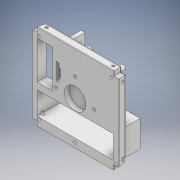
# Autodesk Inventor part: boxbase_solar_esp8285
Saved by Autodesk Inventor 2017 (Build 210142000, 142)
## iProperties
Created: 2018-12-11
Part Number: boxbase_solar_esp8285
Material: ABS Plastic
Document SubType Name: Modeling
Designer: simulator
Density: 1.06 g/cm^3
Appearance: Smooth - White
Mass: 72.9733 g
Surface Area: 351.505 cm^2
Volume: 68.8428 cm^3
Author: simulator
## iProperties of the stored document boxbase_solar_esp8285_3DPrint.ipt
Created: 2019-04-02
Part Number: boxbase_solar_esp8285_3DPrint
Material: Generic
Document SubType Name: Modeling
Designer: simulator
Density: 1 g/cm^3
Appearance: Default
Author: simulator
Autodesk Inventor part; units mm, degrees
ref_plane "YZ Plane" through (0, 0, 0) normal (1, 0, 0) x (0, 1, 0)
sketch "Sketch1" plane through (0, 0, 0) normal (0, 1, 0) x (-1, 0, 0)
  circle A0 centre (45, -45) radius 1.5
  circle A1 centre (-45, 45) radius 1.5
  circle A2 centre (-45, -45) radius 1.5
  circle A3 centre (45, 45) radius 1.5
  line L0 (-50, -50) -> (50, -50)
  line L1 (50, 50) -> (50, -50)
  line L2 (-50, 50) -> (50, 50)
  line L3 (-50, -50) -> (-50, 50)
  line L4 (40, -45) -> (-40, -45)
  line L5 (-40, -40) -> (-40, -45)
  line L6 (-45, -40) -> (-40, -40)
  line L7 (-45, -40) -> (-45, 40)
  line L8 (-40, 40) -> (-45, 40)
  line L9 (-40, 45) -> (-40, 40)
  line L10 (-40, 45) -> (40, 45)
  line L11 (40, 40) -> (40, 45)
  line L12 (45, 40) -> (40, 40)
  line L13 (45, 40) -> (45, -40)
  line L14 (40, -40) -> (45, -40)
  line L15 (40, -45) -> (40, -40)
  point P0 (0, 0)
  point P1 (0, 0)
  constraints: 32 end point, 4 centre point
extrude "Extrusion1" add sketch "Sketch1" along normal blind 10 contours L4 L5 L6 L7 L8 L9 L10 L11 L12 L13 L14 L15
sketch "Sketch2" plane through (45, 0, 40) normal (1, 0, 0) x (0, 0, -1)
  line L0 (0, 10) -> (80, 10)
  line L1 (0, 0) -> (0, 10)
  line L2 (0, 0) -> (80, 0)
  line L3 (80, 10) -> (80, 0)
  circle A0 centre (5, 5) radius 1.5
  circle A1 centre (75, 5) radius 1.5
  point P0 (40, 0)
  point P1 (40, 0)
  constraints: 8 end point, 2 centre point, 2 coincident
hole "Hole1" at (45, 5, 35) at (45, 5, -35) direction (-1, 0, 0) diameter 3 depth 8 tip angle 118
sketch "Sketch3" plane through (-40, 0, 45) normal (0, 0, 1) x (1, 0, 0)
  line L0 (0, 10) -> (80, 10)
  line L1 (0, 0) -> (0, 10)
  line L2 (0, 0) -> (80, 0)
  line L3 (80, 10) -> (80, 0)
  circle A0 centre (5, 5) radius 1.5
  circle A1 centre (75, 5) radius 1.5
  point P0 (40, 0)
  point P1 (40, 0)
  constraints: 8 end point, 2 centre point, 2 coincident
hole "Hole2" at (-35, 5, 45) at (35, 5, 45) direction (0, 0, -1) diameter 3 depth 8 tip angle 118
sketch "Sketch4" plane through (0, 10, 0) normal (0, 1, 0) x (1, 0, 0)
  point P0 (0, 0)
sketch "Sketch5" plane through (40, 0, -45) normal (0, 0, -1) x (-1, 0, 0)
  line L0 (0, 10) -> (80, 10)
  line L1 (0, 0) -> (0, 10)
  line L2 (0, 0) -> (80, 0)
  line L3 (80, 10) -> (80, 0)
  circle A0 centre (5, 5) radius 1.5
  circle A1 centre (75, 5) radius 1.5
  circle A2 centre (75, 5) radius 1.5 projected
  point P0 (40, 0)
  point P1 (40, 0)
  constraints: 8 end point, 2 centre point, 2 coincident
hole "Hole3" at (-35, 5, -45) at (35, 5, -45) direction (0, 0, 1) diameter 3 depth 8 tip angle 118
sketch "Sketch6" plane through (-45, 0, -40) normal (-1, 0, 0) x (0, 0, 1)
  line L0 (0, 10) -> (80, 10)
  line L1 (0, 0) -> (0, 10)
  line L2 (0, 0) -> (80, 0)
  line L3 (80, 10) -> (80, 0)
  circle A0 centre (5, 5) radius 1.5
  circle A1 centre (75, 5) radius 1.5
  circle A2 centre (5, 5) radius 1.5 projected
  circle A3 centre (75, 5) radius 1.5 projected
  point P0 (40, 0)
  point P1 (40, 0)
  constraints: 8 end point, 2 centre point, 2 coincident
hole "Hole4" at (-45, 5, -35) at (-45, 5, 35) direction (1, 0, 0) diameter 3 depth 8 tip angle 118
chamfer "Chamfer1" distance 1 distance2 9 1 edges at (45, 10, 0)
chamfer "Chamfer2" distance 1 distance2 9 1 edges at (42, 10, 40) measured on face at (42, 10, 39.5)
chamfer "Chamfer3" distance 1 distance2 9 2 edges at (40, 10, 39.5) (40, 10, 42.5) measured on face at (39.5, 10, 42.5) measured on face at (39.5, 10, 39.5)
chamfer "Chamfer4" distance 1 distance2 9 1 edges at (-0.5, 10, 45)
chamfer "Chamfer5" distance 1 distance2 9 1 edges at (-40, 10, 42) measured on face at (-39.5, 10, 42)
chamfer "Chamfer6" distance 1 distance2 9 2 edges at (-39.5, 10, 40) (-42.5, 10, 40) measured on face at (-39.5, 10, 39.5) measured on face at (-42.5, 10, 39.5)
chamfer "Chamfer7" distance 1 distance2 9 1 edges at (-45, 10, -0.5)
chamfer "Chamfer8" distance 1 distance2 9 1 edges at (-42, 10, -40) measured on face at (-42, 10, -39.5)
chamfer "Chamfer9" distance 1 distance2 9 2 edges at (-40, 10, -39.5) (-40, 10, -42.5) measured on face at (-39.5, 10, -39.5) measured on face at (-39.5, 10, -42.5)
chamfer "Chamfer10" distance 1 distance2 9 1 edges at (0.5, 10, -45)
chamfer "Chamfer11" distance 1 distance2 9 1 edges at (40, 10, -42) measured on face at (39.5, 10, -42)
chamfer "Chamfer12" distance 1 distance2 9 2 edges at (39.5, 10, -40) (42, 10, -40) measured on face at (42, 10, -39.5) measured on face at (39.5, 10, -39.5)
sketch "Sketch21" plane through (0, 0, 0) normal (0, -1, 0) x (1, 0, 0)
  line L0 (-40, 36) -> (40, 36)
  line L1 (40, 36) -> (40, 12)
  line L2 (40, 12) -> (-40, 12)
  line L3 (-40, 12) -> (-40, 36)
  point P0 (0, 0)
  dimension "d153" = 80
  dimension "d154" = 24
  dimension "d155" = 40
  dimension "d156" = 12
  constraints: 8 end point, 2 parallel, 1 horizontal
  measures "d153" distance of L1.end L2.end
  measures "d154" distance of L0.end L1.end
  measures "d155" distance from line of L1 point (0, 0)
  measures "d156" distance from line of L2 point (0, 0)
sketch "Sketch24" plane through (0, 10, 0) normal (0, 1, 0) x (1, 0, 0)
  line L0 (28.9892, 33.853) -> (-5.0108, 33.853)
  line L1 (-5.0108, 33.853) -> (-5.0108, -0.147)
  line L2 (-5.0108, -0.147) -> (28.9892, -0.147)
  line L3 (28.9892, -0.147) -> (28.9892, 33.853)
  line L4 (32.9892, 37.853) -> (-9.0108, 37.853)
  line L5 (-9.0108, 37.853) -> (-9.0108, -4.147)
  line L6 (-9.0108, -4.147) -> (32.9892, -4.147)
  line L7 (32.9892, -4.147) -> (32.9892, 37.853)
  line L8 (35, -4) -> (1, -4)
  line L9 (1, -4) -> (1, -38)
  line L10 (1, -38) -> (35, -38)
  line L11 (35, -38) -> (35, -4)
  line L12 (-19.3264, -7.8069) -> (-37.3264, -7.8069)
  line L13 (-37.3264, -7.8069) -> (-37.3264, -32.8069)
  line L14 (-37.3264, -32.8069) -> (-19.3264, -32.8069)
  line L15 (-19.3264, -32.8069) -> (-19.3264, -7.8069)
  line L16 (-34.8264, -7.8069) -> (-21.8264, -7.8069)
  line L17 (44, 39) -> (44, -39) projected
  line L18 (39, -44) -> (-39, -44) projected
  line L19 (45, -40) -> (45, 40) projected
  line L20 (-40, -45) -> (40, -45) projected
  circle A0 centre (1, -4) radius 3
  circle A1 centre (35, -4) radius 3
  circle A2 centre (1, -38) radius 3
  circle A3 centre (35, -38) radius 3
  point P0 (0, 0)
  dimension "d169" = 34
  dimension "d170" = 34
  dimension "d171" = 42
  dimension "d172" = 34
  dimension "d173" = 34
  dimension "d174" = 18
  dimension "d175" = 25
  dimension "d176" = 13
  dimension "d177" = 2.5
  dimension "d215" = 10
  dimension "d216" = 7
  dimension "d217" = 6
  dimension "d218" = 6
  dimension "d219" = 6
  dimension "d220" = 6
  constraints: 34 end point, 10 coincident, 8 parallel, 4 centre point, 4 perpendicular, 3 horizontal, 2 point on line, 3 other
  measures "d169" distance of L2.end L1.end
  measures "d170" distance of L1.end L0.end
  measures "d171" distance of L6.end L4.start
  measures "d172" distance of L10.end L9.end
  measures "d173" distance of L9.end L8.end
  measures "d174" distance of L14.end L13.end
  measures "d175" distance of L13.end L12.end
  measures "d176" distance of L16.start L16.end
  measures "d177" distance from line of L15 L16.end
  measures "d215" distance between parallel lines of L11 L19
  measures "d216" distance between parallel lines of L10 L20
  measures "d217" diameter of A0
  measures "d218" diameter of A1
  measures "d219" diameter of A2
  measures "d220" diameter of A3
sketch "Sketch25" plane through (0, 10, 0) normal (0, 1, 0) x (1, 0, 0)
  line L0 (-40, 36) -> (40, 36)
  line L1 (40, 36) -> (40, 12)
  line L2 (40, 12) -> (-40, 12)
  line L3 (-40, 12) -> (-40, 36)
  line L4 (42, 10) -> (42, 38)
  line L5 (42, 38) -> (-42, 38)
  line L6 (-42, 38) -> (-42, 10)
  line L7 (-42, 10) -> (42, 10)
  point P0 (0, 0)
  point P1 (0, 0)
  dimension "d178" = 80
  dimension "d179" = 24
  dimension "d180" = 40
  dimension "d181" = 12
  dimension "d182" = 2
  constraints: 16 end point, 4 parallel, 1 horizontal, 3 other
  measures "d178" distance of L1.end L2.end
  measures "d179" distance of L0.end L1.end
  measures "d180" distance from line of L1 point (0, 0)
  measures "d181" distance from line of L2 point (0, 0)
  measures "d182" distance between parallel lines of L1 L4
extrude "Extrusion19" add sketch "Sketch25" along normal blind 14
sketch "Sketch26" plane through (0, 24, 0) normal (0, 1, 0) x (1, 0, 0)
  line L0 (40, 36) -> (40, 12) projected
  line L1 (42, 10) -> (42, 38) projected
  line L2 (40, 36) -> (40, 12) projected
  line L3 (40, 12) -> (-40, 12) projected
  line L4 (-40, 12) -> (-40, 36) projected
  line L5 (-40, 36) -> (40, 36) projected
  line L6 (42, 10) -> (42, 38) projected
  line L7 (42, 38) -> (-42, 38) projected
  line L8 (-42, 38) -> (-42, 10) projected
  line L9 (-42, 10) -> (42, 10) projected
  point P0 (0, 0)
extrude "Extrusion20" add sketch "Sketch26" along normal blind 2 contours L0 L3 L4 L5 | L9 L8 L7 L1
sketch "Sketch27" plane through (0, 0, 0) normal (0, -1, 0) x (1, 0, 0)
  line L0 (40, -36) -> (40, -12) projected
  line L1 (40, -12) -> (-40, -12) projected
  line L2 (-40, -36) -> (40, -36) projected
  line L3 (-40, -12) -> (-40, -36) projected
  point P0 (0, 0)
extrude "Extrusion21" cut sketch "Sketch27" against normal blind 24
sketch "Sketch28" plane through (0, 26, 0) normal (0, 1, 0) x (1, 0, 0)
  line L0 (-37, 33) -> (-12, 33)
  line L1 (-12, 33) -> (-12, 15)
  line L2 (-12, 15) -> (-37, 15)
  line L3 (-37, 15) -> (-37, 33)
  line L4 (-12, 17.5) -> (-12, 30.5)
  line L5 (-42, 38) -> (-42, 10) projected
  line L6 (42, 38) -> (-42, 38) projected
  circle A0 centre (-12, 30.5) radius 3
  circle A1 centre (-12, 17.5) radius 3
  line L7 (0, 36.4802) -> (32, 36.4802)
  line L8 (32, 36.4802) -> (32, 4.4802)
  line L9 (32, 4.4802) -> (0, 4.4802)
  line L10 (0, 4.4802) -> (0, 36.4802)
  point P0 (0, 0)
  dimension "d189" = 25
  dimension "d190" = 18
  dimension "d191" = 13
  dimension "d192" = 2.5
  dimension "d193" = 5
  dimension "d194" = 5
  dimension "d195" = 6
  dimension "d196" = 6
  dimension "d213" = 32
  dimension "d214" = 32
  constraints: 18 end point, 4 coincident, 4 parallel, 2 centre point, 2 horizontal, 2 perpendicular, 2 point on line
  measures "d189" distance of L1.end L2.end
  measures "d190" distance of L0.end L1.end
  measures "d191" distance of L4.start L4.end
  measures "d192" distance of L4.start L1.end
  measures "d193" distance between parallel lines of L5 L3
  measures "d194" distance between parallel lines of L6 L0
  measures "d195" diameter of A0
  measures "d196" diameter of A1
  measures "d213" distance of L8.end L9.end
  measures "d214" distance of L7.end L8.end
extrude "Extrusion22" add sketch "Sketch28" along normal blind 5 contours A0 L1 L0 | L0 L1 A0 | A1 L1 L2 | L2 L1 A1
sketch "Sketch29" plane through (-12, 31, -17.5) normal (0, 1, 0) x (1, 0, 0)
  circle A0 centre (0, 13) radius 3 projected
  circle A1 centre (0, 0) radius 3 projected
  point P0 (12, -17.5)
  constraints: 2 coincident
hole "Hole6" at (-12, 31, -17.5) at (-12, 31, -30.5) direction (0, -1, 0) diameter 3 depth 8 tip angle 118
sketch "Sketch30" plane through (0, 26, 0) normal (0, 1, 0) x (1, 0, 0)
  circle A0 centre (-12, 17.5) radius 3 projected
  circle A1 centre (-12, 30.5) radius 3 projected
  line L0 (42, 10) -> (42, 38) projected
  line L1 (42, 38) -> (-42, 38) projected
  line L2 (-42, 38) -> (-42, 10) projected
  line L3 (-42, 10) -> (42, 10) projected
  line L4 (42, 10) -> (42, 38) projected
  line L5 (-42, 10) -> (42, 38)
  point P0 (0, 0)
  point P1 (0, 24)
  constraints: 2 end point, 1 midpoint
hole "Hole7" at (0, 26, -24) direction (0, -1, 0) diameter 3 depth 8 tip angle 118
extrude "Extrusion23" add sketch "Sketch24" along normal blind 5 contours A1 L11 L8 L7 | L7 L8 A1 | L8 L11 A1 L6 L7 | L7 L6 A1 L8 | A0 L8 L9 L6 | L6 L9 A0 | A0 L6 L9 L8 | L6 A0 L9 | A3 L10 L11 | L11 L10 A3 | A2 L10 L9 | L9 L10 A2
sketch "Sketch31" plane through (1, 15, 4) normal (0, 1, 0) x (1, 0, 0)
  circle A0 centre (0, 0) radius 3 projected
  circle A1 centre (34, 0) radius 3 projected
  circle A2 centre (0, -34) radius 3 projected
  circle A3 centre (34, -34) radius 3 projected
  circle A4 centre (0, 0) radius 3 projected
  circle A5 centre (34, 0) radius 3 projected
  point P0 (-1, 4)
  constraints: 4 coincident
hole "Hole8" at (1, 15, 4) at (1, 15, 38) at (35, 15, 38) at (35, 15, 4) direction (0, -1, 0) diameter 3 depth 8 tip angle 118
sketch "Sketch32" plane through (0, 10, 0) normal (0, 1, 0) x (1, 0, 0)
  line L0 (-30, 2) -> (-25, 2)
  line L1 (-25, 2) -> (-25, -30)
  line L2 (-25, -30) -> (-30, -30)
  line L3 (-30, -30) -> (-30, 2)
  line L4 (-45, 40) -> (-45, -40) projected
  line L5 (-40, -45) -> (40, -45) projected
  point P0 (0, 0)
  dimension "d230" = 5
  dimension "d231" = 32
  dimension "d232" = 15
  dimension "d233" = 15
  constraints: 8 end point, 2 parallel, 1 horizontal, 1 perpendicular
  measures "d230" distance of L1.end L2.end
  measures "d231" distance of L0.end L1.end
  measures "d232" distance between parallel lines of L3 L4
  measures "d233" distance between parallel lines of L2 L5
ref_plane "Work Plane1" through (-25, 10, 30) normal (1, 0, 0) x (0, 0, -1)
sketch "Sketch35" plane through (0, 10, 0) normal (0, 1, 0) x (1, 0, 0)
  line L0 (42, 10) -> (-42, 10) projected
  line L1 (-42, 10) -> (-42, 38) projected
  line L2 (-42, 38) -> (42, 38) projected
  line L3 (42, 38) -> (42, 10) projected
  line L4 (39, 39) -> (44, 39) projected
  line L5 (39, 44) -> (39, 39) projected
  line L6 (-39, 44) -> (39, 44) projected
  line L7 (-39, 39) -> (-39, 44) projected
  line L8 (-44, 39) -> (-39, 39) projected
  line L9 (-44, -39) -> (-44, 39) projected
  line L10 (-39, -39) -> (-44, -39) projected
  line L11 (-39, -44) -> (-39, -39) projected
  line L12 (39, -44) -> (-39, -44) projected
  line L13 (39, -39) -> (39, -44) projected
  line L14 (44, -39) -> (39, -39) projected
  line L15 (44, 39) -> (44, -39) projected
  circle A0 centre (1, -38) radius 3 projected
  circle A1 centre (1, -4) radius 3 projected
  circle A2 centre (35, -4) radius 3 projected
  circle A3 centre (35, -38) radius 3 projected
  circle A4 centre (0, 4) radius 4
  point P0 (0, 0)
  dimension "d244" = 8
  dimension "d245" = 4
  constraints: 1 centre point
  measures "d244" diameter of A4
  measures "d245" distance of A4.centre point (0, 0)
ref_plane "Work Plane2" through (0, 60, -4) normal (0, 1, 0) x (1, 0, 0)
sketch "Sketch37" plane through (0, 0, 0) normal (0, -1, 0) x (1, 0, 0)
  circle A0 centre (0, 0) radius 11.25
  dimension "d256" = 22.5
  constraints: 1 centre point, 1 coincident
  measures "d256" diameter of A0
extrude "Extrusion28" cut sketch "Sketch37" against normal blind 5
sketch "Sketch38" plane through (0, 0, 0) normal (0, -1, 0) x (1, 0, 0)
  circle A0 centre (0, 0) radius 11.25 projected
  line L0 (-40, -12) -> (40, -12) projected
  line L1 (40, -12) -> (40, -36) projected
  line L2 (40, -36) -> (-40, -36) projected
  line L3 (-40, -36) -> (-40, -12) projected
  line L4 (45, -40) -> (40, -40) projected
  line L5 (45, 40) -> (45, -40) projected
  line L6 (40, 40) -> (45, 40) projected
  line L7 (40, 45) -> (40, 40) projected
  line L8 (-40, 45) -> (40, 45) projected
  line L9 (-40, 40) -> (-40, 45) projected
  line L10 (-45, 40) -> (-40, 40) projected
  line L11 (-45, -40) -> (-45, 40) projected
  line L12 (-40, -40) -> (-45, -40) projected
  line L13 (-40, -45) -> (-40, -40) projected
  line L14 (40, -45) -> (-40, -45) projected
  line L15 (40, -40) -> (40, -45) projected
  point P0 (0, 0)
sketch "Sketch39" plane through (0, 0, 0) normal (0, -1, 0) x (1, 0, 0)
  line L0 (-30, -2) -> (-38, -2)
  line L1 (-38, -2) -> (-38, 30)
  line L2 (-38, 30) -> (-30, 30)
  circle A0 centre (0, 0) radius 11.25
  line L3 (-45, -40) -> (-45, 40)
  line L4 (40, -40) -> (40, -45)
  line L5 (40, -45) -> (-40, -45)
  line L6 (40, -36) -> (-40, -36)
  line L7 (-40, -12) -> (40, -12)
  line L8 (-40, 45) -> (40, 45)
  line L9 (45, -40) -> (40, -40)
  line L10 (40, 45) -> (40, 40)
  line L11 (45, 40) -> (45, -40)
  line L12 (40, 40) -> (45, 40)
  line L13 (40, -12) -> (40, -36)
  line L14 (-40, -45) -> (-40, -40)
  line L15 (-40, -40) -> (-45, -40)
  line L16 (-40, -36) -> (-40, -12)
  line L17 (-30, 30) -> (-30, -2)
  line L18 (-40, 40) -> (-40, 45)
  line L19 (-45, 40) -> (-40, 40)
  circle A1 centre (0, 0) radius 14
  line L20 (0, 0) -> (0, 20)
  circle A2 centre (0, 20) radius 4
  line L21 (0, 0) -> (20, 0)
  line L22 (0, 0) -> (-20, 0)
  circle A3 centre (20, 0) radius 4
  circle A4 centre (-20, 0) radius 4
  line L23 (42, -10) -> (-42, -10)
  line L24 (-42, -10) -> (-42, -38)
  line L25 (-42, -38) -> (42, -38)
  line L26 (42, -38) -> (42, -10)
  line L27 (4, 20) -> (20, 4)
  line L28 (24, 0) -> (42, -10)
  line L29 (-4, 20) -> (-20, 4)
  line L30 (-24, 0) -> (-42, -10)
  circle A5 centre (0, -40) radius 4
  point P0 (0, 0)
  point P1 (0, 0)
  point P2 (0, 0)
  dimension "d259" = 28
  dimension "d260" = 20
  dimension "d261" = 8
  dimension "d262" = 20
  dimension "d263" = 20
  dimension "d264" = 8
  dimension "d265" = 8
  dimension "d266" = 2
  dimension "d267" = 8
  dimension "d268" = 2
  constraints: 62 end point, 9 coincident, 6 centre point, 6 point on circle, 4 horizontal, 3 vertical, 2 point on line, 1 perpendicular, 4 other
  measures "d259" diameter of A1
  measures "d260" distance of L21.start L20.end
  measures "d261" diameter of A2
  measures "d262" distance of L21.start L21.end
  measures "d263" distance of L21.start L22.end
  measures "d264" diameter of A3
  measures "d265" diameter of A4
  measures "d266" distance between parallel lines of L7 L23
  measures "d267" diameter of A5
  measures "d268" distance from line of L25 A5.centre
hole "Hole10" at (-20, 0, 0) at (0, 0, 20) at (20, 0, 0) at (0, 0, -40) direction (0, 1, 0) diameter 3 depth 15 tip angle 118
sketch "Sketch42" plane through (0, 10, 0) normal (0, 1, 0) x (1, 0, 0)
  line L0 (-24, 5) -> (-40, 5)
  line L1 (-40, 5) -> (-40, -35)
  line L2 (-40, -35) -> (-24, -35)
  line L3 (-24, -35) -> (-24, 5)
  line L4 (-45, 40) -> (-45, -40) projected
  line L5 (-40, -45) -> (40, -45) projected
  point P0 (0, 0)
  dimension "d298" = 16
  dimension "d299" = 40
  dimension "d300" = 5
  dimension "d301" = 10
  constraints: 8 end point, 2 parallel, 1 horizontal, 1 perpendicular
  measures "d298" distance of L2.end L1.end
  measures "d299" distance of L1.end L0.end
  measures "d300" distance between parallel lines of L1 L4
  measures "d301" distance between parallel lines of L2 L5
extrude "Extrusion31" cut sketch "Sketch42" against normal blind 40
sketch "Sketch43" plane through (0, 10, 0) normal (0, 1, 0) x (1, 0, 0)
  line L0 (-24, 5) -> (-24, -35) projected
  line L1 (-24, 5) -> (-20, 5)
  line L2 (-20, 5) -> (-20, -35)
  line L3 (-20, -35) -> (-24, -35)
  line L4 (-24, -35) -> (-24, 5)
  point P0 (0, 0)
  dimension "d304" = 4
  constraints: 8 end point, 2 parallel, 1 horizontal, 1 perpendicular
  measures "d304" distance of L2.end L3.end
extrude "Extrusion32" add sketch "Sketch43" along normal blind 20
sketch "Sketch44" plane through (-24, 0, -5) normal (-1, 0, 0) x (0, 0, 1)
  line L0 (40, 0) -> (0, 0) projected
  line L1 (40, 10) -> (40, 0) projected
  line L2 (40, 10) -> (40, 30) projected
  line L3 (0, 30) -> (40, 30) projected
  line L4 (0, 10) -> (0, 30) projected
  line L5 (0, 10) -> (0, 0) projected
  line L6 (0, 25) -> (40, 25)
  point P0 (5, 0)
  point P1 (7.5, 25)
  point P2 (20, 25)
  point P3 (32.5, 25)
  dimension "d307" = 5
  dimension "d308" = 7.5
  dimension "d309" = 7.5
  constraints: 4 point on line, 2 end point, 1 midpoint, 1 perpendicular
  measures "d307" distance between parallel lines of L3 L6
  measures "d308" distance from line of L4 point (7.5, 25)
  measures "d309" distance from line of point (32.5, 25) L2
hole "Hole11" at (-24, 25, 2.5) at (-24, 25, 15) at (-24, 25, 27.5) direction (1, 0, 0) diameter 3 depth 8 tip angle 118
sketch "Sketch48" plane through (0, 10, 0) normal (0, 1, 0) x (1, 0, 0)
  line L0 (-43, -38) -> (-43, 38)
  line L1 (-43, -38) -> (-43, 38)
  line L2 (-43, 38) -> (-38, 38)
  line L3 (-38, 38) -> (-38, 43)
  line L4 (-38, 43) -> (38, 43)
  line L5 (38, 43) -> (38, 38)
  line L6 (38, 38) -> (43, 38)
  line L7 (43, 38) -> (43, -38)
  line L8 (43, -38) -> (38, -38)
  line L9 (38, -38) -> (38, -43)
  line L10 (38, -43) -> (-38, -43)
  line L11 (-38, -43) -> (-38, -38)
  line L12 (-38, -38) -> (-43, -38)
  line L13 (-39, 39) -> (-44, 39)
  line L14 (-44, 39) -> (-44, -39)
  line L15 (-44, -39) -> (-39, -39)
  line L16 (-39, -39) -> (-39, -44)
  line L17 (-39, -44) -> (39, -44)
  line L18 (39, -44) -> (39, -39)
  line L19 (39, -39) -> (44, -39)
  line L20 (44, -39) -> (44, 39)
  line L21 (44, 39) -> (39, 39)
  line L22 (39, 39) -> (39, 44)
  line L23 (39, 44) -> (-39, 44)
  line L24 (-39, 44) -> (-39, 39)
  line L25 (70.5084, 72.789) -> (-67.2775, 72.789)
  line L26 (-67.2775, 72.789) -> (-67.2775, -63.0964)
  line L27 (-67.2775, -63.0964) -> (70.5084, -63.0964)
  line L28 (70.5084, -63.0964) -> (70.5084, 72.789)
  point P0 (0, 0)
  point P1 (0, 0)
  constraints: 58 end point, 2 parallel, 1 horizontal, 1 perpendicular
extrude "Extrusion35" cut sketch "Sketch48" against normal blind 2 contours L24 L23 L22 L21 L20 L19 L18 L17 L16 L15 L14 L13 | L28 L27 L26 L25
sketch "Sketch49" plane through (0, 10, 0) normal (0, 1, 0) x (1, 0, 0)
  line L0 (38, -38) -> (43, -38) projected
  line L1 (38, -43) -> (38, -38) projected
  line L2 (38, 38) -> (38, 43) projected
  line L3 (43, 38) -> (42, 38) projected
  line L4 (-38, 43) -> (-38, 38) projected
  line L5 (-43, -38) -> (-38, -38) projected
  point P0 (0, 0)
  constraints: 4 coincident
hole "Hole12" at (-38, 10, 38) at (38, 10, 38) at (43, 10, -38) at (-38, 10, -38) direction (0, -1, 0) diameter 3 depth 50 tip angle 118
pattern_linear "Rectangular Pattern1" count 2 spacing 40 along (1, 0, 0) of "Extrusion22", "Hole6"
sketch "Sketch50" plane through (0, 26, 0) normal (0, 1, 0) x (1, 0, 0)
  line L0 (40, 36) -> (40, 12) projected
  circle A0 centre (28, 17.5) radius 3 projected
  circle A1 centre (28, 30.5) radius 3 projected
  circle A2 centre (0, 24) radius 1.5 projected
  circle A3 centre (-12, 17.5) radius 3 projected
  circle A4 centre (-12, 30.5) radius 3 projected
  line L1 (42, 10) -> (42, 38) projected
  line L2 (42, 38) -> (-42, 38) projected
  line L3 (-42, 38) -> (-42, 10) projected
  line L4 (-42, 10) -> (42, 10) projected
  circle A5 centre (38, 24) radius 1.5
  circle A6 centre (-38, 24) radius 1.5
  point P0 (0, 0)
  dimension "d337" = 3
  dimension "d338" = 3
  dimension "d339" = 4
  dimension "d340" = 4
  constraints: 2 centre point
  measures "d337" diameter of A5
  measures "d338" diameter of A6
  measures "d339" distance from line of A6.centre L3
  measures "d340" distance from line of L1 A5.centre
extrude "Extrusion36" cut sketch "Sketch50" against normal blind 10 contours A5 | A6
sketch "Sketch51" plane through (0, 10, 0) normal (0, 1, 0) x (1, 0, 0)
  line L0 (-20, -1.5) -> (-20, -35) projected
  line L1 (-20, 5) -> (-20, 1.5) projected
  line L2 (-20, -35) -> (-20, -15)
  line L3 (-17, -6) -> (-20, -6)
  line L4 (-20, -6) -> (-20, -24)
  line L5 (-20, -24) -> (-17, -24)
  line L6 (-17, -24) -> (-17, -6)
  line L7 (-20, -24) -> (-16, -24)
  line L8 (-16, -24) -> (-16, -6)
  line L9 (-16, -6) -> (-20, -6)
  line L10 (-20, -6) -> (-20, -24)
  line L11 (-20, -35) -> (-20, 5) projected
  point P0 (0, 0)
  point P1 (-20, -15)
  dimension "d344" = 20
  dimension "d345" = 3
  dimension "d346" = 18
  dimension "d349" = 4
  dimension "d350" = 18
  constraints: 18 end point, 4 parallel, 3 midpoint, 2 horizontal, 2 perpendicular, 1 point on line
  measures "d344" distance of L2.end L0.end
  measures "d345" distance of L5.end L4.end
  measures "d346" distance of L4.end L3.end
  measures "d349" distance of L9.end L8.end
  measures "d350" distance of L8.end L7.end
extrude "Extrusion37" cut sketch "Sketch51" against normal through all contours L3 L6 L5 L0
sketch "Sketch53" plane through (0, 0, 0) normal (0, -1, 0) x (1, 0, 0)
  line L0 (-20, 6) -> (-20, 24) projected
  line L1 (-15.5, 19.25) -> (-20, 19.25)
  line L2 (-20, 19.25) -> (-20, 10.75)
  line L3 (-20, 10.75) -> (-15.5, 10.75)
  line L4 (-15.5, 10.75) -> (-15.5, 19.25)
  point P0 (0, 0)
  point P1 (-20, 15)
  dimension "d353" = 4.5
  dimension "d354" = 8.5
  constraints: 8 end point, 2 midpoint, 2 parallel, 1 horizontal, 1 perpendicular
  measures "d353" distance of L3.end L2.end
  measures "d354" distance of L2.end L1.end
extrude "Extrusion39" cut sketch "Sketch53" against normal blind 4
body "Solid1"
